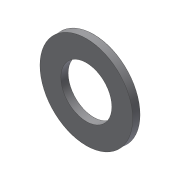
# Autodesk Inventor part: 90945A710_NAS620C5L_flat_washer
Saved by Autodesk Inventor 2014 SP1 (Build 180222100, 222)
## iProperties
Created: 2019-06-26
Part Number: 90945A710_NAS620C5L_flat_washer
Material: Generic
Document SubType Name: Modeling
Designer: RDavis
Density: 1 g/cm^3
Appearance: Default
Author: RDavis
Autodesk Inventor part; units mm, degrees
ref_plane "YZ Plane" through (0, 0, 0) normal (1, 0, 0) x (0, 1, 0)
ref_plane "XZ Plane" through (0, 0, 0) normal (0, 1, 0) x (-1, 0, 0)
ref_plane "XY Plane" through (0, 0, 0) normal (0, 0, 1) x (1, 0, 0)
sketch "Sketch1" plane through (0, 0, 0) normal (0, 0, 1) x (1, 0, 0)
  circle A0 centre (0, 0) radius 1.4605
  circle A1 centre (0, 0) radius 2.6543
  dimension "d0" = 2.921
  dimension "d1" = 5.3086
  constraints: 2 centre point, 2 coincident
  measures "d0" diameter of A0
  measures "d1" diameter of A1
extrude "Extrusion1" add sketch "Sketch1" along normal mid plane 0.4191
body "Solid1"
